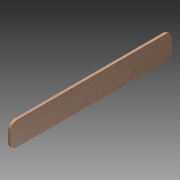
# Autodesk Inventor part: Bumper Wood Backing Part2 (24x28 robot)
Saved by Autodesk Inventor 2013 (Build 170138000, 138)
## iProperties
Created: 2013-01-06
Part Number: Bumper Wood Backing Part2 (24x28 robot)
Material: Wood (Birch)
Document SubType Name: Modeling
Designer: Moses
Density: 0.55 g/cm^3
Mass: 669.303 g
Surface Area: 2134.94 cm^2
Volume: 1216.91 cm^3
Author: Moses
Autodesk Inventor part; units mm, degrees
ref_plane "YZ Plane" through (0, 0, 0) normal (1, 0, 0) x (0, 1, 0)
ref_plane "XZ Plane" through (0, 0, 0) normal (0, 1, 0) x (-1, 0, 0)
ref_plane "XY Plane" through (0, 0, 0) normal (0, 0, 1) x (1, 0, 0)
sketch "Sketch1" plane through (0, 0, 0) normal (0, 0, 1) x (1, 0, 0)
  line L0 (0, 0) -> (0, 127)
  line L1 (0, 127) -> (12.7, 127)
  line L2 (12.7, 127) -> (12.7, 0)
  line L3 (12.7, 0) -> (0, 0)
  dimension "d0" = 127
  dimension "d1" = 12.7
  constraints: 8 end point, 2 parallel, 1 perpendicular, 1 vertical
  measures "d0" distance of L0.start L0.end
  measures "d1" distance of L0.end L1.end
extrude "Extrusion1" add sketch "Sketch1" along normal blind 863.6
fillet "Fillet1" radius 33.3375 4 edges at (6.35, 127, 863.6) (6.35, 0, 863.6) (6.35, 127, 0) (6.35, 0, 0)
body "Solid1"
